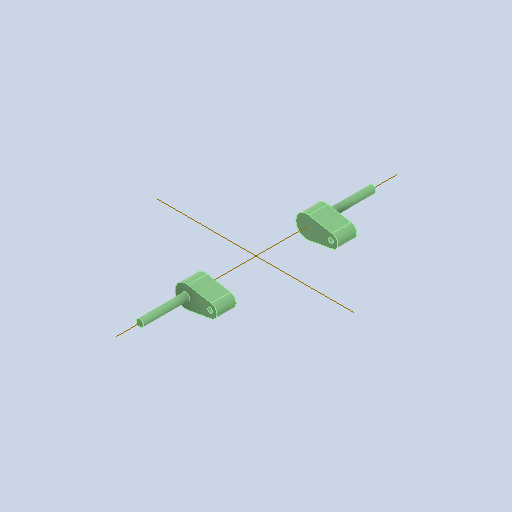
# Autodesk Inventor part: Type 1A R2延伸曲柄:1
Saved by Autodesk Inventor 2025 (Build 290162000, 162)
## iProperties
Created: 2024-09-21
Part Number: Type 1A R2延伸曲柄:1
Material: 密度7850的鋼
Document SubType Name: Modeling
Designer: veter
Density: 7.84999 g/cm^3
Appearance: 平滑 - 深森林綠
Mass: 37500 g
Surface Area: 2777.63 cm^2
Volume: 4777.07 cm^3
Stock Number: 2
Author: veter
Autodesk Inventor part; units mm, degrees
ref_plane "YZ Plane" through (0, 0, 0) normal (1, 0, 0) x (0, 1, 0)
ref_plane "XZ Plane" through (0, 0, 0) normal (0, 1, 0) x (-1, 0, 0)
ref_plane "工作平面2" through (0, 0, 378) normal (0, 0, 1) x (1, 0, 0)
sketch "草圖1" plane through (189, 0, 378) normal (0, 0, 1) x (0, 1, 0)
  line L0 (0, 189) -> (0, 59) construction
  line L1 (-59.0945, 178.6154) -> (-36.9341, 52.5096)
  line L2 (36.9341, 52.5096) -> (59.0945, 178.6154)
  arc A0 (59.0945, 178.6154) -> (-59.0945, 178.6154) centre (0, 189) ccw
  arc A1 (-36.9341, 52.5096) -> (36.9341, 52.5096) centre (0, 59) ccw
  point P0 (0, 124)
  dimension "d1" = 130
  dimension "d2" = 60
  dimension "d3" = 37.5
  constraints: 8 end point, 4 point on circle, 4 tangent, 2 centre point, 1 midpoint, 1 vertical
  measures "d1" distance of L0.start L0.end
  measures "d2" radius of A0
  measures "d3" radius of A1
extrude "擠出1" add sketch "草圖1" against normal blind 103
sketch "草圖2" plane through (189, 0, 378) normal (0, 0, 1) x (1, 0, 0)
  circle A0 centre (-189, 0) radius 19.875
  dimension "d6" = 39.75
  constraints: 1 centre point, 1 coincident
  measures "d6" diameter of A0
extrude "擠出2" add sketch "草圖2" along normal blind 250
sketch "草圖3" plane through (189, 0, 378) normal (0, 0, 1) x (1, 0, 0)
  arc A0 (-52.5096, -36.9341) -> (-52.5096, 36.9341) centre (-59, 0) ccw projected
  circle A1 centre (-59, 0) radius 13.25
  point P0 (-189, 0)
  dimension "d9" = 26.5
  constraints: 1 centre point, 1 coincident
  measures "d9" diameter of A1
extrude "擠出3" cut sketch "草圖3" against normal through all
sketch "草圖4" plane through (136.4904, 36.9341, 275) normal (0.1730769, 0.9849083, 0) x (0, 0, 1)
  line L0 (103, 0) -> (0, 0) projected
  point P0 (-275, -128.0381)
  point P1 (51.5, 0)
  constraints: 1 midpoint
hole "孔1" [suppressed]
sketch "草圖5" plane through (10.3846, -59.0945, 275) normal (0.1730769, -0.9849083, 0) x (0.9849083, 0.1730769, 0)
  line L0 (128.0381, 103) -> (128.0381, 0) projected
  point P0 (0, -275)
  point P1 (128.0381, 51.5)
  constraints: 1 midpoint
hole "孔2" [suppressed]
mirror "鏡射2" about plane through (0, 0, 0) normal (0, 0, 1) of "擠出1", "擠出2", "擠出3"
equation "\"d1\" = R2"
equation "\"R2\" = T1A_R2"
equation "\"Width\" = T1A_R2_Width"
equation "\"d19\" = 0.5 * Width"
equation "\"T1A_R2_Width\" = 756"
equation "\"T1A_R1\" = 585.5331"
equation "\"T1A_R3\" = 252.3048"
equation "\"T1A_R4\" = 320.6953"
equation "\"T1A_R5\" = 419.3047"
equation "\"T1A_R7\" = -221.7475"
equation "\"T1A_R8\" = 369.2781"
equation "\"T1A_R1_Width\" = 756"
equation "\"T1A_R3_Width\" = 344"
equation "\"T1A_R4_Width\" = 756"
equation "\"T1A_Joint_Width\" = 756"
equation "\"T1A_R2\" = 130"
